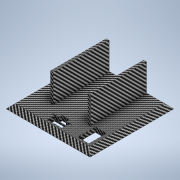
# Autodesk Inventor part: Base Plate
Saved by Autodesk Inventor 2021.1 (Build 251245010, 245A)
## iProperties
Created: 2020-11-23
Part Number: Base Plate
Material: CFRP
Document SubType Name: Modeling
Designer: elizh
Density: 1.43 g/cm^3
Appearance: Carbon Fiber
Author: elizh
Autodesk Inventor part; units mm, degrees
ref_plane "YZ Plane" through (0, 0, 0) normal (1, 0, 0) x (0, 1, 0)
ref_plane "XZ Plane" through (0, 0, 0) normal (0, 1, 0) x (-1, 0, 0)
ref_plane "XY Plane" through (0, 0, 0) normal (0, 0, 1) x (1, 0, 0)
sketch "Sketch1" plane through (0, 0, 0) normal (0, 1, 0) x (-1, 0, 0)
  line L0 (45, 45) -> (-45, 45)
  line L1 (-45, 45) -> (-45, -45)
  line L2 (-45, -45) -> (45, -45)
  line L3 (45, -45) -> (45, 45)
  line L4 (0, 0) -> (55.2623, 0) construction
  line L5 (0, 0) -> (0, -72.148) construction
  dimension "d0" = 90
  constraints: 12 end point, 2 horizontal, 2 parallel, 2 perpendicular, 1 vertical, 2 other
  measures "d0" distance of L2.end L0.start
extrude "Extrusion1" add sketch "Sketch1" along normal blind 5
chamfer "Chamfer2" distance 5 angle 45 4 edges at (-45, 5, 0) (0, 5, -45) (45, 5, 0) (0, 5, 45)
sketch "Sketch5" plane through (0, 5, 0) normal (0, 1, 0) x (1, 0, 0)
  line L0 (-7.75, -30.5) -> (7.75, -30.5)
  line L1 (7.75, -30.5) -> (7.75, -38)
  line L2 (7.75, -38) -> (-7.75, -38)
  line L3 (-7.75, -38) -> (-7.75, -30.5)
  line L4 (0, 0) -> (0, 19.274) construction
  line L5 (-3.75, -26) -> (3.75, -26)
  line L6 (3.75, -26) -> (3.75, -29.5)
  line L7 (3.75, -29.5) -> (-3.75, -29.5)
  line L8 (-3.75, -29.5) -> (-3.75, -26)
  line L9 (40, -40) -> (-40, -40) projected
  dimension "d13" = 15.5
  dimension "d14" = 7.5
  dimension "d15" = 1
  dimension "d16" = 7.5
  dimension "d17" = 3.5
  dimension "d18" = 2
  constraints: 18 end point, 4 parallel, 2 horizontal, 2 perpendicular, 1 vertical, 2 other
  measures "d13" distance of L0.start L0.end
  measures "d14" distance of L0.end L1.end
  measures "d15" distance between parallel lines of L0 L7
  measures "d16" distance of L5.start L5.end
  measures "d17" distance of L5.end L6.end
  measures "d18" distance between parallel lines of L9 L2
extrude "Extrusion3" cut sketch "Sketch5" against normal through all
sketch "Sketch6" plane through (0, 5, 0) normal (0, 1, 0) x (1, 0, 0)
  line L0 (-7.75, -30.5) -> (7.75, -30.5) construction
  line L1 (3.75, -29.5) -> (-3.75, -29.5) construction
  line L2 (-10.5, -29.5) -> (10.5, -29.5)
  line L3 (10.5, -29.5) -> (10.5, -30.5)
  line L4 (10.5, -30.5) -> (-10.5, -30.5)
  line L5 (-10.5, -30.5) -> (-10.5, -29.5)
  line L6 (0, 0) -> (0, 31.4057) construction
  dimension "d21" = 21
  constraints: 10 end point, 2 collinear, 2 parallel, 1 horizontal, 1 perpendicular, 1 vertical, 1 other
  measures "d21" distance of L2.start L2.end
extrude "Extrusion4" cut sketch "Sketch6" against normal blind 4
sketch "Sketch7" plane through (0, 5, 0) normal (0, 1, 0) x (1, 0, 0)
  line L0 (-18.5, 39) -> (18.5, 39) construction
  line L1 (-3.75, -26) -> (3.75, -26) projected
  line L2 (-18.5, 39) -> (-18.5, -21)
  line L3 (18.5, 39) -> (18.5, -21)
  line L4 (-18.5, -21) -> (18.5, -21) construction
  line L5 (0, 0) -> (0, 26.3141) construction
  line L6 (18.5, -21) -> (21.5, -21)
  line L7 (21.5, -21) -> (21.5, 39)
  line L8 (21.5, 39) -> (18.5, 39)
  line L9 (-18.5, 39) -> (-21.5, 39)
  line L10 (-21.5, 39) -> (-21.5, -21)
  line L11 (-21.5, -21) -> (-18.5, -21)
  dimension "d24" = 65
  dimension "d25" = 5
  dimension "d26" = 37
  dimension "d27" = 3
  dimension "d28" = 3
  constraints: 22 end point, 4 perpendicular, 3 horizontal, 3 vertical, 2 point on line, 1 other
  measures "d24" distance between parallel lines of L1 L0
  measures "d25" distance between parallel lines of L1 L4
  measures "d26" distance of L2.end L3.end
  measures "d27" distance of L7.end L0.end
  measures "d28" distance of L0.start L9.end
extrude "Extrusion5" add sketch "Sketch7" along normal blind 30
sketch "Sketch8" plane through (0, 5, 0) normal (0, 1, 0) x (1, 0, 0)
  line L0 (24.75, -19) -> (36.75, -19)
  line L1 (36.75, -19) -> (36.75, -38)
  line L2 (36.75, -38) -> (24.75, -38)
  line L3 (24.75, -38) -> (24.75, -19)
  line L4 (40, 40) -> (40, -40) projected
  line L5 (21.5, -21) -> (21.5, 39) projected
  line L6 (7.75, -38) -> (-7.75, -38) projected
  point P0 (0, 0)
  dimension "d31" = 19
  dimension "d32" = 12
  dimension "d33" = 18.5
  dimension "d34" = 3.25
  constraints: 8 end point, 2 parallel, 1 collinear, 1 horizontal, 1 perpendicular
  measures "d31" distance of L0.end L1.end
  measures "d32" distance of L0.start L0.end
  measures "d33" distance between parallel lines of L4 L5
  measures "d34" distance between parallel lines of L4 L1
extrude "Extrusion6" cut sketch "Sketch8" against normal through all
equation "\"d28\" = d27"
equation "\"d34\" = -0.5 * d32 + 0.5 * d33"
body "Solid1"
